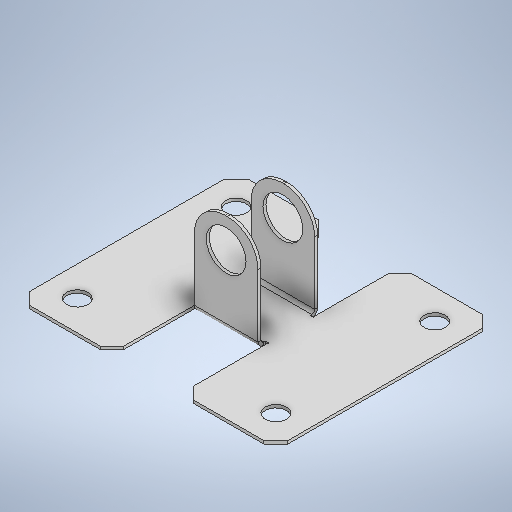
# Autodesk Inventor part: Piston_floor_hinge
Saved by Autodesk Inventor 2025.2 (Build 292293000, 293)
## iProperties
Created: 2025-04-29
Part Number: Piston_floor_hinge
Material: Generic
Document SubType Name: Sheet Metal
Designer: Caspe
Density: 1 g/cm^3
Sheet Metal Rule: Default_mm
Appearance: Default
Flat Pattern Width: 13 cm
Flat Pattern Length: 12.4786 cm
Flat Pattern Area: 162.222 cm^2
Sheet Metal Width: 130,000 mm
Sheet Metal Length: 124,786 mm
Sheet Metal Area: 16222,159 mm^2
Author: Caspe
Autodesk Inventor part; units mm, degrees
ref_plane "YZ Plane" through (0, 0, 0) normal (1, 0, 0) x (0, 1, 0)
ref_plane "XZ Plane" through (0, 0, 0) normal (0, 1, 0) x (-1, 0, 0)
ref_plane "XY Plane" through (0, 0, 0) normal (0, 0, 1) x (1, 0, 0)
sketch "Sketch1" plane through (0, 0, 0) normal (0, 1, 0) x (-1, 0, 0)
  line L0 (0, 0) -> (-130, 0)
  line L1 (-130, 0) -> (-130, -110)
  line L2 (-130, -110) -> (0, -110)
  line L3 (0, -110) -> (0, 0)
  circle A0 centre (-15, -15) radius 5.35
  line L4 (-65, -110) -> (-65, 0)
  line L5 (0, -55) -> (-130, -55)
  circle A1 centre (-115, -15) radius 5.35
  circle A2 centre (-15, -95) radius 5.35
  circle A3 centre (-115, -95) radius 5.35
  line L6 (-47.5, -110) -> (-82.5, -110)
  line L7 (-82.5, -110) -> (-82.5, -68.5)
  line L8 (-82.5, -68.5) -> (-47.5, -68.5)
  line L9 (-47.5, -68.5) -> (-47.5, -110)
  line L10 (-82.5, 0) -> (-82.5, -41.5)
  line L11 (-82.5, -41.5) -> (-47.5, -41.5)
  line L12 (-47.5, -41.5) -> (-47.5, 0)
  dimension "d0" = 130
  dimension "d1" = 110
  dimension "d2" = 10.7
  dimension "d3" = 100
  dimension "d4" = 80
  dimension "d5" = 35
  dimension "d6" = 35
  dimension "d7" = 27
  measures "d0" distance of L2.end L1.end
  measures "d1" distance of L1.end L0.end
  measures "d2" diameter of A0
  measures "d3" diameter of A0.centre L4
  measures "d4" diameter of A0.centre L5
  measures "d5" diameter of L9 L4
  measures "d6" diameter of L7 L4
  measures "d7" diameter of L8 L5
extrude "Plate1" add sketch "Sketch1" along normal blind 1.5 contours L3 L5 L4 L11 L12 L0 | L3 L2 L9 L8 L4 L5 | L5 L1 L0 L10 L11 L4 | L4 L8 L7 L2 L1 L5
sketch "Sketch2" plane through (82.5, 0, -40) normal (0, 0, -1) x (-1, 0, 0)
  line L0 (33.5, 0) -> (1.5, 0)
  line L1 (1.5, 0) -> (1.5, 50)
  line L2 (1.5, 50) -> (33.5, 50)
  line L3 (33.5, 50) -> (33.5, 0)
  constraints: 8 end point
edge flange "Flange1" height 50 angle 90 thickness 1.5 bend radius 1.5 thickness toward (0, 0, -1) relief straight relief width 1.5 relief depth 0.75 corner gap 1.5 corner form 0 edges at (65, 1.5, -41.5) (65, 1.5, -68.5) wall of the first edge with corners at (49, 0, -40) (81, 0, -40) (81, 50, -40) (49, 50, -40)
bend "Bend1"
corner "Corner1"
sketch "Sketch3" plane through (49, 50, -40) normal (0, 0, 1) x (1, 0, 0)
  line L0 (32, 0) -> (0, 0) projected
  line L1 (16, 0) -> (16, -78.39)
  circle A0 centre (16, -15) radius 10
  point P0 (-49, -50)
  dimension "d19" = 20
  dimension "d20" = 15
  constraints: 2 end point, 1 centre point, 1 midpoint, 1 point on line, 1 vertical
  measures "d19" diameter of A0
  measures "d20" distance from line of L0 A0.centre
fillet "Corner Round1" radius 15.5 4 edges at (49, 50, -40.75) (81, 50, -40.75) (81, 50, -69.25) (49, 50, -69.25)
extrude "Cut1" cut sketch "Sketch3" against normal up to surface (30 mm away)
chamfer "Corner Chamfer1" distance 6 angle 45 8 edges at (0, 0.75, 0) (47.5, 0.75, 0) (82.5, 0.75, 0) (130, 0.75, 0) (130, 0.75, -110) (82.5, 0.75, -110) (47.5, 0.75, -110) (0, 0.75, -110)
equation "\"d6\" = d5"
equation "\"d22\" = Thickness"
equation "\"d8\" = Thickness"
equation "\"d9\" = BendReliefWidth"
equation "\"d10\" = BendReliefDepth"
equation "\"d11\" = MinimumRemnant"
equation "\"d12\" = TransitionRadius"
equation "\"d15\" = BendRadius"
equation "\"d16\" = CornerReliefSize"
equation "\"d17\" = GapSize"
equation "\"d18\" = JacobiRadiusSize"
equation "\"Thickness\" = plate_thickness"
equation "\"BendRadius\" = Thickness"
equation "\"BendReliefWidth\" = Thickness"
equation "\"BendReliefDepth\" = 0.5 * Thickness"
equation "\"CornerReliefSize\" = 4 * Thickness"
equation "\"MinimumRemnant\" = 2 * Thickness"
equation "\"TransitionRadius\" = BendRadius"
equation "\"JacobiRadiusSize\" = BendRadius"
equation "\"GapSize\" = Thickness"
equation "\"A_joint_diameter\" = 16"
equation "\"A_B_spacing\" = 2"
equation "\"A_joint_tolerance\" = 3"
equation "\"l___________\" = 0"
equation "\"l__________\" = 0"
equation "\"l_________\" = 0"
equation "\"rivet_diameter\" = 3.35"
equation "\"plate_thickness\" = 1.5"
equation "\"l________\" = 0"
equation "\"L_Piston_Top\" = 25"
equation "\"L_Piston_Bottom\" = 21"
body "Solid1"
